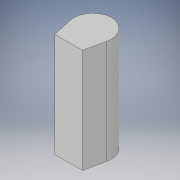
# Autodesk Inventor part: JlinearActuator
Saved by Autodesk Inventor 2018 (Build 220112000, 112)
## iProperties
Created: 2020-04-10
Part Number: JlinearActuator
Material: Generic
Document SubType Name: Modeling
Designer: Jesse R-B
Density: 1 g/cm^3
Appearance: Default
Author: Jesse R-B
Autodesk Inventor part; units mm, degrees
ref_plane "YZ Plane" through (0, 0, 0) normal (1, 0, 0) x (0, 1, 0)
ref_plane "XZ Plane" through (0, 0, 0) normal (0, 1, 0) x (-1, 0, 0)
ref_plane "XY Plane" through (0, 0, 0) normal (0, 0, 1) x (1, 0, 0)
sketch "Sketch1" plane through (0, 0, 0) normal (0, 1, 0) x (-1, 0, 0)
  arc A0 (8.4455, 23.8147) -> (8.3223, 23.1255) centre (8.7463, 23.4053) ccw construction
  arc A1 (8.4455, 23.8147) -> (14.6473, 39.363) centre (0.0001, 36.1944) ccw construction
  line L0 (14.6473, 39.363) -> (11.148, 55.5389) construction
  arc A2 (11.5371, 56.1429) -> (11.148, 55.5389) centre (11.6445, 55.6463) ccw construction
  line L1 (11.5371, 56.1429) -> (13.5232, 56.5725) construction
  arc A3 (14.1273, 56.1832) -> (13.5232, 56.5725) centre (13.6307, 56.076) ccw construction
  line L2 (14.1273, 56.1832) -> (17.6265, 40.0078) construction
  arc A4 (10.1518, 21.2894) -> (17.6265, 40.0078) centre (0.0002, 36.1948) ccw construction
  arc A5 (9.4419, 21.4294) -> (10.1518, 21.2894) centre (9.8658, 21.7093) ccw construction
  line L3 (9.4419, 21.4294) -> (8.3223, 23.1255) construction
  arc A6 (-13.5232, 56.5725) -> (-14.1271, 56.1834) centre (-13.6306, 56.076) ccw construction
  line L4 (-13.5232, 56.5725) -> (-11.5371, 56.1429) construction
  arc A7 (-11.148, 55.5389) -> (-11.5371, 56.1429) centre (-11.6445, 55.6463) ccw construction
  line L5 (-11.148, 55.5389) -> (-14.6472, 39.3636) construction
  arc A8 (-14.6472, 39.3636) -> (-8.4594, 23.8249) centre (0, 36.195) ccw construction
  arc A9 (-8.3222, 23.1257) -> (-8.4594, 23.8249) centre (-8.7461, 23.4056) ccw construction
  line L6 (-8.3222, 23.1257) -> (-9.4417, 21.4297) construction
  arc A10 (-10.1516, 21.2896) -> (-9.4417, 21.4297) centre (-9.8656, 21.7095) ccw construction
  arc A11 (-17.6263, 40.0081) -> (-10.1516, 21.2896) centre (0, 36.195) ccw construction
  line L7 (-17.6263, 40.0081) -> (-14.1271, 56.1834) construction
  line L8 (11.148, 55.5389) -> (14.6473, 39.363)
  arc A12 (8.4455, 23.8147) -> (14.6473, 39.363) centre (0.0001, 36.1944) ccw
  line L9 (-11.148, 55.5389) -> (-14.6472, 39.3636)
  arc A13 (-14.6472, 39.3636) -> (-8.4594, 23.8249) centre (0, 36.195) ccw
  line L10 (11.148, 55.5389) -> (-11.148, 55.5389)
  arc A14 (-8.4594, 23.8249) -> (8.4455, 23.8147) centre (0, 35.3068) ccw
  point P0 (0, 0)
  constraints: 30 point on circle, 22 end point, 15 centre point, 5 tangent, 1 concentric, 1 horizontal
extrude "Extrusion1" add sketch "Sketch1" along normal blind 83.82
body "Solid1"
